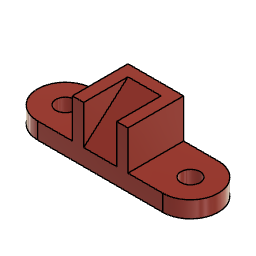
Exercise 2 (Autodesk Fusion 360 design; units mm, degrees)
Autodesk Fusion 360 part; units mm, degrees
sketch "Sketch1" plane through (0, 0, 0) normal (0, 0, 1) x (1, 0, 0)
  line L0 (0, 0) -> (144, 0)
  line L1 (144, 64) -> (0, 64)
  circle A0 centre (144, 32) radius 11
  circle A1 centre (0, 32) radius 11
  arc A2 (0, 64) -> (0, 0) centre (0, 32) ccw
  arc A3 (144, 0) -> (144, 64) centre (144, 32) ccw
  constraint coincident L0.start A2.end
  constraint horizontal L0
  constraint concentric A0 A3
  constraint coincident L0 A2.end
extrude "Extrude1" add sketch "Sketch1" along normal blind 19
sketch "Sketch2" plane through (0, 0, 19) normal (0, 0, 1) x (-1, 0, 0)
  circle A0 centre (-144, -32) radius 11
  circle A1 centre (0, -32) radius 11
  arc A2 (-144, 0) -> (-144, -64) centre (-144, -32) ccw
  line L0 (-144, -64) -> (0, -64)
  arc A3 (0, -64) -> (0, 0) centre (0, -32) ccw
  line L1 (0, 0) -> (-144, 0)
  line L2 (-72, -64) -> (-104, -64)
  line L3 (-104, -64) -> (-104, 0)
  line L4 (-104, 0) -> (-91, 0)
  line L5 (-91, 0) -> (-91, -51)
  line L6 (-91, -51) -> (-72, -51)
  line L7 (-40, 0) -> (-53, 0)
  line L8 (-53, 0) -> (-53, -51)
  line L9 (-53, -51) -> (-72, -51)
  line L10 (-72, -64) -> (-40, -64)
  line L11 (-40, -64) -> (-40, 0)
  dimension "d7" = 32
  dimension "d8" = 13
  dimension "d9" = 51
  constraint midpoint L0 L2.start
  constraint coincident L1 L3.end
  constraint perpendicular L1 L3
  constraint perpendicular L3 L4
  constraint perpendicular L1 L5
  measures "d7" distance of L2.start L2.end
  measures "d8" distance of L3.end L4.end
  measures "d9" distance of L4.end L5.end
extrude "Extrude2" add sketch "Sketch2" along normal blind 45 contours L0 L1 L2 L3 L4 L5 L6 L7 L8 L9 L10 L11
sketch "Sketch3" plane through (53, 0, 0) normal (1, 0, 0) x (0, 1, 0)
  line L0 (0, 19) -> (51, 19)
  line L1 (51, 19) -> (51, 64)
  line L2 (51, 64) -> (0, 64)
  line L3 (0, 64) -> (0, 19)
  line L4 (0, 19) -> (51, 64)
  line L5 (51, 64) -> (51, 19)
  line L6 (0, 19) -> (51, 19)
  constraint coincident L0.start L3.end
  constraint coincident L1.end L2.start
  constraint coincident L0.end L1.start
extrude "Extrude3" add sketch "Sketch3" along normal blind 50 contours L0 L1 L4 L5 L6
